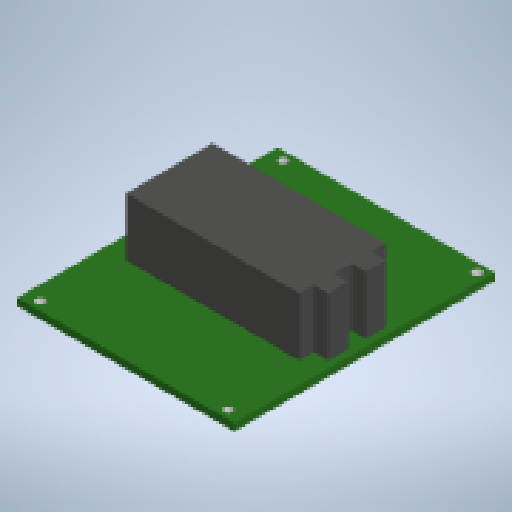
# Autodesk Inventor part: control_board
Saved by Autodesk Inventor 2024.1 (Build 281209000, 209)
## iProperties
Created: 2024-08-02
Part Number: control_board
Material: 一般
Document SubType Name: Modeling
Designer: hibik
Density: 1 g/cm^3
Appearance: 既定
Author: hibik
Autodesk Inventor part; units mm, degrees
ref_plane "YZ Plane" through (0, 0, 0) normal (1, 0, 0) x (0, 1, 0)
ref_plane "XZ Plane" through (0, 0, 0) normal (0, 1, 0) x (-1, 0, 0)
ref_plane "XY Plane" through (0, 0, 0) normal (0, 0, 1) x (1, 0, 0)
sketch "スケッチ1" plane through (0, 0, 0) normal (0, 1, 0) x (-1, 0, 0)
  line L0 (0, 0) -> (75, 0)
  line L1 (75, 0) -> (75, -90)
  line L2 (75, -90) -> (0, -90)
  line L3 (0, -90) -> (0, 0)
  circle A0 centre (70, -3) radius 1.5
  circle A1 centre (70, -87) radius 1.5
  circle A2 centre (5, -3) radius 1.5
  circle A3 centre (5, -87) radius 1.5
  dimension "d0" = 75
  dimension "d1" = 90
  dimension "d4" = 3
  dimension "d5" = 5
  dimension "d6" = 3
  dimension "d7" = 3
  dimension "d8" = 5
  dimension "d9" = 5
  dimension "d10" = 3
  dimension "d11" = 3
  constraints: 8 end point, 4 centre point, 3 equal radius, 2 parallel, 1 horizontal, 1 perpendicular, 1 vertical alignment
  measures "d0" distance of L1.end L2.end
  measures "d1" distance of L0.end L1.end
  measures "d4" diameter of A0
  measures "d5" distance from line of L1 A0.centre
  measures "d6" distance from line of L0 A0.centre
  measures "d7" distance from line of L2 A1.centre
  measures "d8" distance from line of L1 A1.centre
  measures "d9" distance from line of L3 A2.centre
  measures "d10" distance from line of L0 A2.centre
  measures "d11" distance from line of L2 A3.centre
extrude "押し出し1" add sketch "スケッチ1" along normal blind 2.5
sketch "スケッチ2" plane through (0, 2.5, 0) normal (0, 1, 0) x (1, 0, 0)
  line L0 (-67.5, 30) -> (-7.5, 30)
  line L1 (-7.5, 30) -> (-7.5, 60)
  line L2 (-7.5, 60) -> (-67.5, 60)
  line L3 (-67.5, 60) -> (-67.5, 30)
  line L4 (-75, 90) -> (-75, 0) projected
  line L5 (0, 90) -> (-75, 90) projected
  line L6 (-7.5, 35) -> (-2.5, 35)
  line L7 (-2.5, 35) -> (-2.5, 42)
  line L8 (-2.5, 42) -> (-7.5, 42)
  line L9 (-7.5, 42) -> (-7.5, 35)
  line L10 (-7.5, 48) -> (-2.5, 48)
  line L11 (-2.5, 48) -> (-2.5, 55)
  line L12 (-2.5, 55) -> (-7.5, 55)
  line L13 (-7.5, 55) -> (-7.5, 48)
  point P0 (0, 0)
  point P1 (-67.5, 45)
  point P2 (-75, 45)
  point P3 (-37.5, 60)
  point P4 (-37.5, 90)
  dimension "d13" = 30
  dimension "d14" = 60
  dimension "d15" = 5
  dimension "d16" = 5
  dimension "d17" = 7
  dimension "d18" = 5
  constraints: 24 end point, 6 parallel, 4 collinear, 4 midpoint, 3 horizontal, 3 perpendicular, 1 horizontal alignment, 1 vertical alignment
  measures "d13" distance of L2.end L0.start
  measures "d14" distance of L0.start L0.end
  measures "d15" distance between parallel lines of L0 L6
  measures "d16" distance between parallel lines of L2 L12
  measures "d17" distance of L8.end L6.start
  measures "d18" distance between parallel lines of L7 L1
extrude "押し出し2" add sketch "スケッチ2" along normal blind 20
equation "\"d7\" = d6"
equation "\"d9\" = d5"
equation "\"d10\" = d6"
equation "\"d11\" = d6"
equation "\"d16\" = d15"
